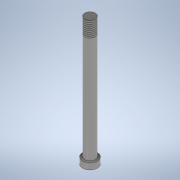
# Autodesk Inventor part: Connector_1
Saved by Autodesk Inventor 2022 (Build 260153000, 153)
## iProperties
Created: 2023-01-17
Part Number: Connector_1
Material: Steel, Mild
Document SubType Name: Modeling
Designer: 48735
Density: 7.85 g/cm^3
Appearance: Semi-Polished
Author: 48735
Autodesk Inventor part; units mm, degrees
ref_plane "YZ Plane" through (0, 0, 0) normal (1, 0, 0) x (0, 1, 0)
ref_plane "XZ Plane" through (0, 0, 0) normal (0, 1, 0) x (-1, 0, 0)
ref_plane "XY Plane" through (0, 0, 0) normal (0, 0, 1) x (1, 0, 0)
sketch "Sketch1" plane through (0, 0, 0) normal (0, 1, 0) x (-1, 0, 0)
  circle A0 centre (0, 0) radius 2.5
  dimension "d0" = 5
  constraints: 1 centre point, 1 coincident
  measures "d0" diameter of A0
extrude "Extrusion1" add sketch "Sketch1" along normal blind 58
sketch "Sketch2" plane through (0, 0, 0) normal (0, -1, 0) x (1, 0, 0)
  circle A0 centre (0, 0) radius 3.5
  dimension "d3" = 7
  constraints: 1 centre point, 1 coincident
  measures "d3" diameter of A0
extrude "Extrusion2" add sketch "Sketch2" along normal blind 3
thread "Thread1" size "M5x0.8" class "6g" standard "ANSI Metric M Profile" length 7.5
sketch "Sketch3" plane through (0, -3, 0) normal (0, -1, 0) x (1, 0, 0)
  circle A0 centre (0, 0) radius 2.5 projected
  line L0 (1.7236, -1.0145) -> (-0.0168, -1.9999)
  line L1 (-0.0168, -1.9999) -> (-1.7404, -0.9854)
  line L2 (-1.7404, -0.9854) -> (-1.7236, 1.0145)
  line L3 (-1.7236, 1.0145) -> (0.0168, 1.9999)
  line L4 (0.0168, 1.9999) -> (1.7404, 0.9854)
  line L5 (1.7404, 0.9854) -> (1.7236, -1.0145)
  constraints: 12 end point, 1 coincident, 13 other
extrude "Extrusion3" cut sketch "Sketch3" against normal blind 1 contours L0 L1 L2 L3 L4 L5
body "Solid1"
